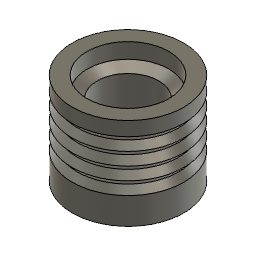
capstan_pulley_ed (Autodesk Fusion 360 design; units mm, degrees)
Autodesk Fusion 360 part; units mm, degrees
sketch "Sketch1" plane through (0, 0, 0) normal (0, 1, 0) x (1, 0, 0)
  circle A0 centre (0, 0) radius 10.936
  dimension "d2" = 21.872
  constraint coincident A0.centre origin
  measures "d2" diameter of A0
extrude "Extrude1" add sketch "Sketch1" along normal mid plane 18
sketch "Sketch2" plane through (0, 9, 0) normal (0, 1, 0) x (-1, 0, 0)
  circle A0 centre (0, 0) radius 10.936
  circle A1 centre (0, 0) radius 8.02
  dimension "d7" = 16.04
  constraint coincident A0.centre A1.centre
  measures "d7" diameter of A1
extrude "Extrude2" cut sketch "Sketch2" against normal blind 18 contours A1
sketch "Sketch3" plane through (0, 0, 0) normal (1, 0, 0) x (0, 0, -1)
  line L0 (-10.936, -9) -> (10.936, -9)
  line L1 (10.936, 9) -> (-10.936, 9)
  line L2 (-10.936, 9) -> (-10.936, -9) construction
  line L3 (-10.936, 0) -> (-10.936, -1.25)
  line L4 (-10.936, 0) -> (-10.936, 1.25)
  line L5 (-10.936, 1.25) -> (-9.936, 0)
  line L6 (-9.936, 0) -> (-10.936, -1.25)
  dimension "d12" = 1.25
  dimension "d13" = 1.25
  dimension "d14" = 1
  constraint coincident L1.end L2.start
  constraint coincident L0.start L2.end
  constraint midpoint L2 L3.start
  constraint parallel L2 L3
  constraint parallel L2 L4
  measures "d12" distance of L3.start L3.end
  measures "d13" distance of L3.start L4.end
  measures "d14" distance of L3.start L5.end
revolve "Revolve1" cut sketch "Sketch3" angle 360 about axis through (0, 1.75, 0) along (0, 1, 0)
pattern_linear "R-Pattern1" count 4 spacing 2.5 along (0, 1, 0) both ways of "Revolve1"
ref_plane "WorkPlane1" through (0, 2, 0) normal (0, 1, 0) x (0, 0, 1)
sketch "Sketch4" plane through (0, 0, 0) normal (0, 0, 1) x (1, 0, 0)
  line L0 (-8.02, 9) -> (8.02, 9)
  line L1 (21.75, 2) -> (0.75, 2)
  line L2 (8.02, -9) -> (-8.02, -9)
  line L3 (8.02, -9) -> (8.02, 9) construction
  line L4 (8.02, 2) -> (8.02, -2)
  line L5 (8.02, 2) -> (8.02, 6)
  line L6 (8.02, 2) -> (6.02, 2) construction
  line L7 (6.02, 2) -> (6.02, -1)
  line L8 (6.02, 2) -> (6.02, 5)
  line L9 (8.02, 6) -> (6.02, 5)
  line L10 (6.02, -1) -> (8.02, -2)
  dimension "d24" = 4
  dimension "d25" = 4
  dimension "d26" = 2
  dimension "d27" = 3
  dimension "d28" = 3
  constraint coincident L2.start L3.start
  constraint coincident L0.end L3.end
  constraint coincident L3 L4.start
  constraint coincident L1 L4.start
  constraint perpendicular L1 L4
  constraint perpendicular L1 L5
  constraint perpendicular L3 L6
  constraint perpendicular L6 L7
  constraint perpendicular L6 L8
  measures "d24" distance of L4.start L4.end
  measures "d25" distance of L4.start L5.end
  measures "d26" distance of L4.start L6.end
  measures "d27" distance of L6.end L7.end
  measures "d28" distance of L6.end L8.end
revolve "Revolve2" add sketch "Sketch4" angle 360 about axis through (0, 1.75, 0) along (0, 1, 0)
equation "base_radii = ( ( 10.936 ) * 2 ) * 1 mm"
equation "d2 = base_radii"
equation "extruded_base = 9.0 mm"
equation "d4 = extruded_base"
equation "top_hole_Radii = ( ( 8.02 ) * 2 ) * 1 mm"
equation "d7 = top_hole_Radii"
equation "d8 = -extruded_base * 2"
equation "revolute_tri_height = 1.0 mm"
equation "revolute_tri_base_one_side = revolute_tri_height * 1.25"
equation "d12 = revolute_tri_base_one_side"
equation "d13 = revolute_tri_base_one_side"
equation "d14 = revolute_tri_height"
equation "rev_in_long_side = 4.00 mm"
equation "rev_in_Short_Side = 3 mm"
equation "rev_in_top_gap = 2.00 mm"
equation "d24 = rev_in_long_side"
equation "d25 = rev_in_long_side"
equation "d26 = rev_in_top_gap"
equation "d27 = rev_in_Short_Side"
equation "d28 = rev_in_Short_Side"
